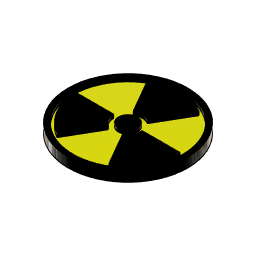
Nuclear Symbol (Autodesk Fusion 360 design; units mm, degrees)
Autodesk Fusion 360 part; units mm, degrees
sketch "Sketch1" plane through (0, 0, 0) normal (0, 0, 1) x (1, 0, 0)
  circle A0 centre (0, 0) radius 25
  dimension "d1" = 50
  constraint coincident A0.centre origin
  measures "d1" diameter of A0
extrude "Extrude1" add sketch "Sketch1" along normal blind 2.5
sketch "Sketch2" plane through (0, 0, 2.5) normal (0, 0, 1) x (-1, 0, 0)
  circle A0 centre (0, 0) radius 25
  circle A1 centre (0, 0) radius 4
  line L0 (-6, 0) -> (-3, -5.1962) construction
  line L1 (-3, -5.1962) -> (3, -5.1962) construction
  line L2 (3, -5.1962) -> (6, 0) construction
  line L3 (6, 0) -> (3, 5.1962) construction
  line L4 (3, 5.1962) -> (-3, 5.1962) construction
  line L5 (-3, 5.1962) -> (-6, 0) construction
  circle A2 centre (0, 0) radius 21.75
  line L6 (-6, 0) -> (-21.75, 0)
  line L7 (6, 0) -> (21.75, 0)
  line L8 (-3, -5.1962) -> (-10.875, -18.8361)
  line L9 (3, -5.1962) -> (10.875, -18.8361)
  line L10 (-10.875, -18.8361) -> (-21.75, 0) construction
  line L11 (10.875, -18.8361) -> (21.75, 0) construction
  line L12 (-3, 5.1962) -> (-10.875, 18.8361)
  line L13 (3, 5.1962) -> (10.875, 18.8361)
  line L14 (10.875, 18.8361) -> (-10.875, 18.8361) construction
  line L15 (-21.75, 0) -> (-10.875, 18.8361) construction
  line L16 (-10.875, -18.8361) -> (10.875, -18.8361) construction
  circle A3 centre (0, 0) radius 6
  circle A4 centre (0, 0) radius 23
  dimension "d4" = 8
  dimension "d5" = 6
  dimension "d6" = 43.5
  dimension "d7" = 46
  constraint concentric A0 A1
  constraint coincident A0.centre A1.centre
  constraint horizontal L4
  constraint concentric A0 A2
  constraint coincident A2 L6.end
  constraint horizontal L6
  constraint coincident A2 L7.end
  constraint horizontal L7
  constraint coincident A2 L8.end
  constraint coincident A2 L9.end
  constraint coincident A2 L12.end
  constraint coincident A2 L13.end
  constraint equal L10 L11
  constraint equal L10 L14
  constraint horizontal L14
  constraint equal L15 L16
  constraint concentric A1 A3
  constraint coincident L0.end A3
  constraint concentric A3 A4
  measures "d4" diameter of A1
  measures "d5" distance of L0.start A0.centre
  measures "d6" diameter of A2
  measures "d7" diameter of A4
extrude "Extrude3" add sketch "Sketch2" along normal blind 1.5 contours A0 | A1 | A2 L7 L13 A3 | A2 L8 L9 A3 | A2 L6 L12 A3
